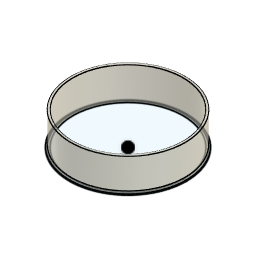
ValveCollar (Autodesk Fusion 360 design; units mm, degrees)
Autodesk Fusion 360 part; units mm, degrees
sketch "Profile" plane through (0, 0, 0) normal (0, 0, 1) x (1, 0, 0)
  circle A0 centre (0, 0) radius 85
  circle A1 centre (0, 0) radius 88
  circle A2 centre (0, 0) radius 90
  dimension "d5" = 170
  dimension "d6" = 3
  dimension "d7" = 5
  constraint coincident A0.centre A1.centre
  measures "d5" diameter of A0
ref_plane "WorkPlane1" through (0, 0, 3.55) normal (0, 0, 1) x (1, 0, 0)
sketch "NegativeFiletProfile" plane through (0, 0, 3.55) normal (0, 0, 1) x (1, 0, 0)
  circle A0 centre (0, 0) radius 90
extrude "Extrude Column" add sketch "Profile" along normal blind 52 contours A1
extrude "Extrude Base" add sketch "Profile" along normal blind 4 contours A2
pipe "Cut Base Filet" cut diameter 4.1 path "NegativeFiletProfile" along A0
fillet "Cut Top Filet" radius 1.5 1 faces at (35.7347, 79.0838, 52)
equation "InnerDiammeter = 170 mm" comment "The inner column the lid passes through"
equation "WallThickness = 3 mm" comment "Thickness of the main wall"
equation "BaseExtension = ( 180 mm - ( InnerDiammeter ) ) / 2" comment "Diameter of outer ring to go under rocks, etc."
equation "BaseHeight = 4 mm" comment "How tall the base should be before flange"
equation "d5 = InnerDiammeter"
equation "d6 = WallThickness"
equation "d7 = BaseExtension"
equation "ColumnHeight = 52 mm" comment "How tall the total extension is from the ground up"
equation "d9 = ColumnHeight"
equation "d11 = BaseHeight"
equation "BaseFiletDiameter = 4.1 mm" comment "Diameter of the inward fillet"
equation "d16 = ( BaseFiletDiameter / 2 ) + BaseFiletOffset"
equation "d19 = BaseFiletDiameter"
equation "BaseFiletOffset = 1.5 mm" comment "How far from the groud does the filet start"
equation "d23 = TopFiletDiameter"
equation "TopFiletDiameter = 1.5 mm" comment "How rounded the top edge is."
named bodies: "ValveCollar"
